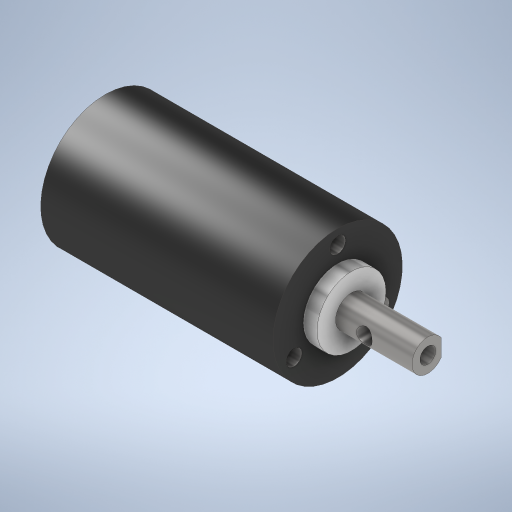
# Autodesk Inventor part: M2006 P36
Saved by Autodesk Inventor 2023 (Build 270158000, 158)
## iProperties
Created: 2023-03-15
Part Number: M2006 P36
Material: ステンレス鋼
Document SubType Name: Modeling
Designer: fhbdh
Density: 8 g/cm^3
Appearance: 半つや出し
Author: fhbdh
Autodesk Inventor part; units mm, degrees
ref_plane "YZ Plane" through (0, 0, 0) normal (1, 0, 0) x (0, 1, 0)
ref_plane "XZ Plane" through (0, 0, 0) normal (0, 1, 0) x (-1, 0, 0)
ref_plane "XY Plane" through (0, 0, 0) normal (0, 0, 1) x (1, 0, 0)
sketch "スケッチ1" plane through (0, 0, 0) normal (1, 0, 0) x (0, 1, 0)
  circle A0 centre (0, 0) radius 12.2
  dimension "d0" = 24.4
  constraints: 1 centre point, 1 coincident
  measures "d0" diameter of A0
extrude "押し出し1" add sketch "スケッチ1" along normal blind 43.8
sketch "スケッチ2" plane through (43.8, 0, 0) normal (1, 0, 0) x (0, 0, -1)
  circle A0 centre (0, 0) radius 6.5
  dimension "d3" = 13
  constraints: 1 centre point, 1 coincident
  measures "d3" diameter of A0
extrude "押し出し2" add sketch "スケッチ2" along normal blind 2.6
sketch "スケッチ3" plane through (46.4, 0, 0) normal (1, 0, 0) x (0, 0, -1)
  circle A0 centre (0, 0) radius 3
  dimension "d6" = 6
  constraints: 1 centre point, 1 coincident
  measures "d6" diameter of A0
extrude "押し出し3" add sketch "スケッチ3" along normal blind 14.4
sketch "スケッチ4" plane through (60.8, 0, 0) normal (1, 0, 0) x (0, 0, -1)
  circle A0 centre (0, 0) radius 3 projected
  line L0 (2.5, 1.6583) -> (2.5, -1.6583)
  line L1 (0, 0) -> (0, -3)
  dimension "d9" = 6
  dimension "d10" = 2.5
  constraints: 4 end point, 3 point on circle, 1 parallel, 1 vertical
  measures "d9" diameter of A0
  measures "d10" distance between parallel lines of L1 L0
extrude "押し出し4" cut sketch "スケッチ4" against normal blind 11.5 contours A0 L0 picked at (2.5914, -0.3806)
sketch "スケッチ5" plane through (60.8, -1.6583, -2.5) normal (0, 0, -1) x (-1, 0, 0)
  line L0 (0, 0) -> (0, 3.3166) projected
  point P0 (60.8, 1.6583)
  point P1 (9, 1.6583)
  point P2 (0, 1.6583)
  dimension "d13" = 0
  dimension "d14" = 9
  constraints: 1 midpoint
  measures "d13" vertical distance of point (0, 1.658) point (9, 1.658)
  measures "d14" distance from line of L0 point (9, 1.658)
hole "穴1" at (51.8, 0, -2.5) direction (0, 0, 1) diameter 3 end through all
sketch "スケッチ6" plane through (0, 0, 0) normal (-1, 0, 0) x (0, 0, 1)
  arc A0 (-2.5, -1.6583) -> (-2.5, 1.6583) centre (0, 0) ccw projected
  circle A1 centre (0, 0) radius 3
  point P0 (-2.5, 1.6583)
  dimension "d22" = 6
  constraints: 1 centre point, 1 coincident
  measures "d22" diameter of A1
extrude "押し出し5" add sketch "スケッチ6" along normal blind 4
sketch "スケッチ7" plane through (60.8, 0, 0) normal (1, 0, 0) x (0, 0, -1)
  circle A0 centre (0, 0) radius 6.5 projected
  circle A1 centre (0, 0) radius 1.5
  dimension "d25" = 3
  constraints: 1 centre point, 1 coincident
  measures "d25" diameter of A1
extrude "押し出し6" cut sketch "スケッチ7" against normal blind 6 contours A1
sketch "スケッチ8" plane through (43.8, 0, 0) normal (1, 0, 0) x (0, 0, -1)
  point P0 (0, 0)
  point P1 (0, 9.5)
  point P2 (-8.2272, -4.75)
  point P3 (8.2272, -4.75)
  dimension "d28" = 0
  dimension "d29" = 9.5
  dimension "d32" = 360
  constraints: 4 other
  measures "d28" horizontal distance of point (0, 0) point (0, 9.5)
  measures "d29" distance of point (0, 0) point (0, 9.5)
hole "穴2" at (43.8, 9.5, 0) at (43.8, -4.75, 8.2272) at (43.8, -4.75, -8.2272) direction (-1, 0, 0) diameter 3 depth 6 tip angle 118
sketch "スケッチ9" plane through (0, 0, 0) normal (-1, 0, 0) x (0, 0, 1)
  point P0 (0, 0)
  point P1 (5.5, 0)
  point P2 (-2.75, 4.7631)
  point P3 (-2.75, -4.7631)
  dimension "d41" = 0
  dimension "d42" = 5.5
  dimension "d45" = 360
  constraints: 4 other
  measures "d41" vertical distance of point (0, 0) point (5.5, 0)
  measures "d42" distance of point (0, 0) point (5.5, 0)
hole "穴3" at (0, 0, 5.5) at (0, 4.7631, -2.75) at (0, -4.7631, -2.75) direction (1, 0, 0) diameter 2 depth 6 tip angle 118
